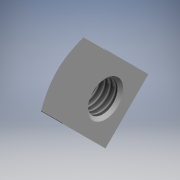
# Autodesk Inventor part: DIN 557 - M10
Saved by Autodesk Inventor 2017.3 (Build 213256000, 256)
## iProperties
Part Number: DIN 557 - M10
Material: Generic
Catalog Web Link: www.cadenas.de
Description: DIN-557-Square nuts
Vendor: FESTO
Document SubType Name: Modeling
Designer: partserver
Manufacturer: FESTO
Mass: 1.82146 g
Surface Area: 11.5554 cm^2
Volume: 1.82146 cm^3
Density: 1 g/cm^3
Appearance: PSOLRGB-192-192-192
Category: PARTsolutions
Company: FESTO
Title: DIN 557 - M10
Author: Cadenas PARTsolutions
Comments: Square nuts
PSOL_IDENT_0: {$CADENAS_DATA\23d-libs\festo\zyl_zubeh\din_557\din_557.prj},180 {VTYP=3D},{NB=DIN 557 - M10},{LINA=
PSOL_IDENT_1: DIN 557 - M10},{NN=DIN-557},{DATE=28.05.2015 11:13:37},{GEOMDATE=10.08.2011 05:48:00},{VERSION=v0706
PSOL_IDENT_2: 19081727},{LINEID=50},{WBVAR=},{WBNUMERIC=}  {NB=DIN 557 - M10},{LINA=DIN 557 - M10},{KT=X},{IDNR=},
PSOL_IDENT_3: {NENN=M10},{D=10.000},{D1=8.376},{P=1.500},{M=8.000},{S=17.000},{SW=},{DW=15.500},{NN=M10}
NB: DIN 557 - M10
NN: M10
NT: Square nuts
NBSYN: DIN 557 - $NENN.
LINA: DIN 557 - M10
CATALOG: Festo
ROWDESC: M10
D: 10
D1: 8.376
P: 1.5
M: 8
S: 17
DW: 15.5
SUPPLIER: FESTO
ARTICLENO: DIN 557 - M10
BOMINFO: DIN 557 - M10
CREATOR: CADENAS GmbH
Autodesk Inventor part; units mm, degrees
sketch "Sketch_2" plane through (0, 0, 0) normal (0, 0, 1) x (1, 0, 0)
  line L0 (8, 0) -> (0, 0)
  line L1 (0, 0) -> (0, 12.0208)
  line L2 (0, 12.0208) -> (6.143, 12.0208)
  line L3 (6.143, 12.0208) -> (8, 7.75)
  line L4 (8, 7.75) -> (8, 0)
  line L5 (8, 0) -> (0, 0)
  constraints: 12 end point
revolve "Revolution1" add sketch "Sketch_2" angle 360 about axis through (8, 0, 0) along (1, 0, 0)
sketch "Skizze_2" plane through (0, 0, 0) normal (1, 0, 0) x (0, 1, 0)
  line L0 (34, 34) -> (-34, 34)
  line L1 (-34, 34) -> (-34, -34)
  line L2 (-34, -34) -> (34, -34)
  line L3 (34, -34) -> (34, 34)
  line L4 (0, 12.0915) -> (-12.0915, 0)
  line L5 (-12.0915, 0) -> (0, -12.0915)
  line L6 (0, -12.0915) -> (12.0915, 0)
  line L7 (12.0915, 0) -> (0, 12.0915)
  constraints: 16 end point
extrude "Extrusion1" cut sketch "Skizze_2" along normal blind 8
sketch "Sketch_1" plane through (0, 0, 0) normal (0, 0, 1) x (1, 0, 0)
  line L0 (8, 0) -> (0, 0)
  line L1 (0, 0) -> (0, 5)
  line L2 (0, 5) -> (0.812, 4.188)
  line L3 (0.812, 4.188) -> (7.188, 4.188)
  line L4 (7.188, 4.188) -> (8, 5)
  line L5 (8, 5) -> (8, 0)
  line L6 (8, 0) -> (0, 0)
  constraints: 14 end point
revolve "Revolution2" cut sketch "Sketch_1" angle 360 about axis through (8, 0, 0) along (1, 0, 0)
thread "Thread1" size "M10x1.5" class "6H" standard "ISO Metric profile" full length
ref_plane "IP1_XY" through (0, 0, 0) normal (1, 0, 0) x (0, 0, -1)
ref_plane "IP1_YZ" through (0, 0, 0) normal (0, 0, -1) x (0, 1, 0)
ref_plane "IP1_ZX" through (0, 0, 0) normal (0, 1, 0) x (1, 0, 0)
ref_plane "IP2_XY" through (8, 0, 0) normal (1, 0, 0) x (0, 0, -1)
ref_plane "IP2_YZ" through (8, 0, 0) normal (0, 0, -1) x (0, 1, 0)
ref_plane "IP2_ZX" through (8, 0, 0) normal (0, 1, 0) x (1, 0, 0)
body "Solid1"
